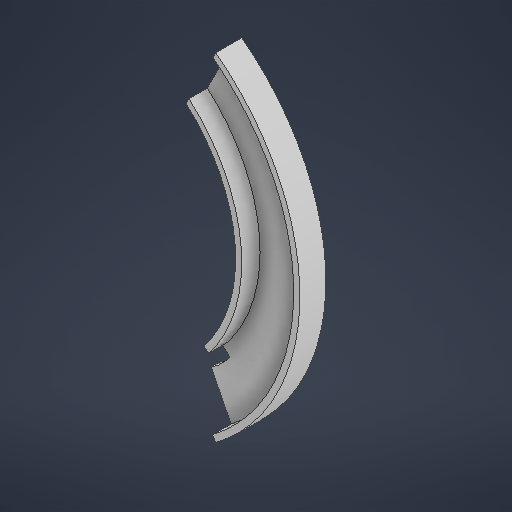
# Autodesk Inventor part: outside3
Saved by Autodesk Inventor 2026.2 (Build 302298000, 298)
## iProperties
Created: 2026-03-14
Part Number: outside3
Material: Generic
Document SubType Name: Modeling
Designer: danda
Density: 1 g/cm^3
Appearance: Default
Author: danda
Autodesk Inventor part; units mm, degrees
ref_plane "YZ Plane" through (0, 0, 0) normal (1, 0, 0) x (0, 1, 0)
ref_plane "XZ Plane" through (0, 0, 0) normal (0, 1, 0) x (-1, 0, 0)
ref_plane "XY Plane" through (0, 0, 0) normal (0, 0, 1) x (1, 0, 0)
sketch "Sketch1" plane through (0, 0, 0) normal (0, 0, 1) x (1, 0, 0)
  arc A0 (967.6192, 924.0732) -> (967.7873, 1075.2272) centre (902.2196, 999.723) ccw
  arc A1 (983.2683, 893.0126) -> (983.4428, 1106.3006) centre (902.2196, 999.723) ccw
  line L0 (965.7611, 927.7614) -> (985.0977, 889.3816)
  line L1 (966.6908, 925.9161) -> (1011.6908, 925.9161) construction
  arc A2 (985.0977, 889.3816) -> (985.2727, 1109.9327) centre (902.2196, 999.723) ccw
  line L2 (965.9281, 1071.5369) -> (985.2727, 1109.9327)
  arc A3 (965.7611, 927.7614) -> (965.9281, 1071.5369) centre (902.2196, 999.723) ccw
  line L3 (977.4986, 940.149) -> (980.6353, 937.6667)
  point P0 (0, 0)
  point P1 (983.9681, 893.1)
  point P2 (990.6031, 1100.4422)
  point P3 (968.1775, 1074.8866)
  dimension "d28" = 100
  dimension "d33" = 63.26
  dimension "d34" = 4
  dimension "d40" = 4
  dimension "d41" = 4
  constraints: 10 point on circle, 8 end point, 5 point on line, 4 centre point, 1 horizontal
  measures "d28" radius of A0
  measures "d33" angle of L0 L1
  measures "d34" radial gap between concentric circles of A1 A2
  measures "d40" radial gap between concentric circles of A0 A3
  measures "d41" distance of L3.start L3.end
extrude "Extrusion6" add sketch "Sketch1" along normal blind 5
extrude "Extrusion7" add sketch "Sketch1" along normal blind 17 contours L3 A3 L2 A0 | A1 L2 A2 L0
sketch "Sketch5" plane through (0, 0, 5) normal (0, 0, 1) x (1, 0, 0)
  arc A0 (965.7611, 927.7614) -> (977.4986, 940.149) centre (902.2196, 999.723) ccw projected
  line L0 (965.7611, 927.7614) -> (970.2605, 918.8308)
  line L1 (965.7611, 927.7614) -> (983.2683, 893.0126) projected
  line L2 (977.4986, 940.149) -> (985.1361, 933.6938)
  arc A1 (965.7611, 927.7614) -> (977.4986, 940.149) centre (902.2196, 999.723) ccw
  arc A2 (965.7611, 927.7614) -> (974.9009, 937.006) centre (902.2196, 999.723) ccw
  line L3 (974.9009, 937.006) -> (982.5384, 930.5509)
  arc A3 (970.2605, 918.8308) -> (982.5384, 930.5509) centre (950.8165, 951.4915) ccw
  point P0 (0, 0)
  dimension "d42" = 10
  dimension "d43" = 10
  dimension "d46" = 13
  dimension "d47" = 10
  constraints: 7 point on circle, 6 end point, 3 centre point, 1 concentric, 1 parallel, 1 point on line
  measures "d42" distance of L0.start L0.end
  measures "d43" distance of L2.start L2.end
  measures "d46" distance of L0.start L3.start
  measures "d47" distance of L3.start L3.end
extrude "Extrusion8" cut sketch "Sketch5" along normal through all both and the other way through all
body "Solid2"
